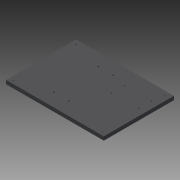
# Autodesk Inventor part: bottom
Saved by Autodesk Inventor 2013 (Build 170138000, 138)
## iProperties
Created: 2013-07-28
Part Number: bottom
Material: Generic
Document SubType Name: Modeling
Designer: employee
Density: 1 g/cm^3
Mass: 979.825 g
Surface Area: 1733.5 cm^2
Volume: 979.825 cm^3
Author: employee
Autodesk Inventor part; units mm, degrees
ref_plane "YZ Plane" through (0, 0, 0) normal (1, 0, 0) x (0, 1, 0)
ref_plane "XZ Plane" through (0, 0, 0) normal (0, 1, 0) x (-1, 0, 0)
ref_plane "XY Plane" through (0, 0, 0) normal (0, 0, 1) x (1, 0, 0)
sketch "Sketch1" plane through (0, 0, 0) normal (0, 0, 1) x (1, 0, 0)
  line L0 (-165.5, 118.75) -> (165.5, 118.75)
  line L1 (165.5, 118.75) -> (165.5, -118.75)
  line L2 (165.5, -118.75) -> (-165.5, -118.75)
  line L3 (-165.5, -118.75) -> (-165.5, 118.75)
  point P0 (0, 0)
  point P1 (-165.5, 0)
  point P2 (0, 118.75)
  dimension "d0" = 331
  dimension "d2" = 237.5
  constraints: 8 end point, 2 midpoint, 2 parallel, 1 horizontal, 1 horizontal alignment, 1 perpendicular, 1 vertical alignment
  measures "d0" distance of L0.start L0.end
  measures "d2" distance of L2.end L0.start
extrude "Extrusion1" add sketch "Sketch1" along normal blind 12.5
sketch "Sketch2" plane through (0, 0, 0) normal (0, 0, -1) x (-1, 0, 0)
  circle A0 centre (-150.5, 103.75) radius 1.55 projected
  line L0 (-145.8379, -108.9576) -> (-147.4259, -106.1413) projected
  circle A1 centre (150.5, -108.75) radius 1.55 projected
  circle A2 centre (150.5, 103.75) radius 1.55 projected
  line L1 (150.5, -108.75) -> (-150.5, -108.75)
  line L2 (-150.5, -108.75) -> (-150.5, 103.75)
  line L3 (-150.5, 103.75) -> (150.5, 103.75)
  line L4 (150.5, 103.75) -> (150.5, -108.75)
  circle A3 centre (-150.5, -108.75) radius 1.55
  point P0 (0, 0)
  constraints: 8 end point, 2 parallel, 1 centre point, 1 coincident, 1 equal radius, 1 horizontal, 1 perpendicular
extrude "Extrusion2" cut sketch "Sketch2" against normal through all contours L3 L2 A0 | A0 L2 L3 | L3 L4 A2 | A2 L4 L3 | A3 L1 L2 | L2 L1 A3 | L4 L1 A1 | A1 L1 L4
sketch "Sketch3" plane through (0, 0, 0) normal (0, 0, -1) x (-1, 0, 0)
  circle A0 centre (150.5, -108.75) radius 1.55
  circle A1 centre (-150.5, 103.75) radius 1.55
  circle A2 centre (-150.5, -108.75) radius 1.55
  circle A3 centre (150.5, 103.75) radius 1.55
  circle A4 centre (-150.5, 103.75) radius 3.25
  circle A5 centre (-150.5, -108.75) radius 3.25
  circle A6 centre (150.5, -108.75) radius 3.25
  circle A7 centre (150.5, 103.75) radius 3.25
  circle A8 centre (-150.5, -108.75) radius 1.55 projected
  point P0 (0, 0)
  dimension "d7" = 6.5
  constraints: 8 centre point, 5 coincident, 3 equal radius
  measures "d7" diameter of A6
hole "Hole1" at (150.5, 103.75, 0) at (150.5, -108.75, 0) at (-150.5, -108.75, 0) at (-150.5, 103.75, 0) direction (0, 0, 1) diameter 3.4 end through all counterbore diameter 6.5 counterbore depth 3 clearance for "Socket Head Cap Screw" size "M3" standard "Ansi Metric M Profile"
sketch "Sketch4" plane through (0, 0, 0) normal (0, 0, -1) x (-1, 0, 0)
  circle A0 centre (-2, -73.75) radius 1.621 projected
  circle A1 centre (48, 76.25) radius 1.621 projected
  circle A2 centre (-2, 76.25) radius 1.621 projected
  circle A3 centre (48, -73.75) radius 1.621 projected
  line L0 (-34.5, 108.75) -> (-34.5, -106.25) projected
  line L1 (-34.5, -106.25) -> (80.5, -106.25) projected
  line L2 (80.5, -106.25) -> (80.5, 108.75) projected
  line L3 (80.5, 108.75) -> (-34.5, 108.75) projected
  point P0 (0, 0)
hole "Hole2" at (-48, -73.75, 0) at (2, -73.75, 0) at (-48, 76.25, 0) at (2, 76.25, 0) direction (0, 0, 1) diameter 4.5 end through all counterbore diameter 8 counterbore depth 4 clearance for "Socket Head Cap Screw" size "M4" standard "Ansi Metric M Profile"
sketch "Sketch5" plane through (0, 0, 0) normal (0, 0, -1) x (-1, 0, 0)
  circle A0 centre (-143.139, 21.4425) radius 1.7 projected
  circle A1 centre (-52.461, 65.2575) radius 1.7 projected
  circle A2 centre (-143.139, 65.2575) radius 1.7 projected
  circle A3 centre (-52.461, 21.4425) radius 1.7 projected
  line L0 (-47, 17.95) -> (-148.6, 17.95) projected
  line L1 (-47, 68.75) -> (-47, 17.95) projected
  line L2 (-148.6, 68.75) -> (-47, 68.75) projected
  line L3 (-148.6, 17.95) -> (-148.6, 68.75) projected
  point P0 (0, 0)
hole "Hole3" at (143.139, 65.2575, 0) at (143.139, 21.4425, 0) at (52.461, 65.2575, 0) at (52.461, 21.4425, 0) direction (0, 0, 1) diameter 3.4 end through all counterbore diameter 6.5 counterbore depth 3 clearance for "Socket Head Cap Screw" size "M3" standard "Ansi Metric M Profile"
body "Solid1"
